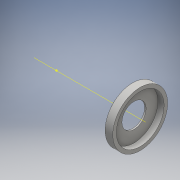
# Autodesk Inventor part: Деталь 4
Saved by Autodesk Inventor 2016 SP1 (Build 200210100, 210)
## iProperties
Created: 2016-05-02
Part Number: Деталь 4
Material: Типовые
Document SubType Name: Modeling
Designer: AS
Density: 1 g/cm^3
Appearance: По умолчанию
Mass: 267.151 g
Surface Area: 826.233 cm^2
Volume: 267.151 cm^3
Author: AS
Autodesk Inventor part; units mm, degrees
ref_plane "YZ Plane" through (0, 0, 0) normal (1, 0, 0) x (0, 1, 0)
ref_plane "XZ Plane" through (0, 0, 0) normal (0, 1, 0) x (-1, 0, 0)
ref_plane "XY Plane" through (0, 0, 0) normal (0, 0, 1) x (1, 0, 0)
sketch "Эскиз1" plane through (0, 0, 0) normal (0, 0, 1) x (1, 0, 0)
  line L0 (258.1011, -41) -> (258.1011, -76)
  line L1 (258.1011, -76) -> (248.1011, -76)
  line L2 (248.1011, -76) -> (248.1011, -81)
  line L3 (248.1011, -81) -> (258.1011, -81)
  line L4 (258.1011, -81) -> (258.1011, -93)
  line L5 (258.1011, -93) -> (284.1011, -93)
  line L6 (284.1011, -93) -> (284.1011, -81)
  line L7 (284.1011, -81) -> (263.1011, -81)
  line L8 (263.1011, -81) -> (263.1011, -41)
  line L9 (263.1011, -41) -> (258.1011, -41)
  line L10 (-56.8202, 0) -> (340.9214, 0) projected
  point P0 (0, 0)
  dimension "d0" = 26
  dimension "d1" = 52
  dimension "d2" = 12
  dimension "d3" = 5
  dimension "d4" = 5
  dimension "d5" = 10
  dimension "d6" = 93
  constraints: 20 end point, 7 perpendicular, 4 point on line, 1 vertical
  measures "d0" distance of L5.end L4.end
  measures "d1" distance between parallel lines of L9 L5
  measures "d2" distance of L3.end L4.end
  measures "d3" distance of L1.end L2.end
  measures "d4" distance of L8.end L0.start
  measures "d5" distance of L2.end L3.end
  measures "d6" distance from line of L5 point (0, 0)
revolve "Вращение1" add sketch "Эскиз1" angle 360 about axis through (-10, 0, 0) along (1, 0, 0)
chamfer "Фаска1" distance 2 angle 45 1 edges at (248.1011, 81, 0)
sketch "Эскиз2" plane through (284.1011, 0, 0) normal (1, 0, 0) x (0, 0, -1)
  point P0 (-87.0155, 0.0233)
  point P1 (-43.4876, 75.3693)
  point P2 (43.5279, 75.346)
  point P3 (87.0155, -0.0233)
  point P4 (43.4876, -75.3693)
  point P5 (-43.5279, -75.346)
hole "Отверстие1" at (284.1011, 0.0233, 87.0155) at (284.1011, 75.3693, 43.4876) at (284.1011, 75.346, -43.5279) at (284.1011, -0.0233, -87.0155) at (284.1011, -75.3693, -43.4876) at (284.1011, -75.346, 43.5279) direction (-1, 0, 0) diameter 5.5 depth 26
